Autodesk Fusion 360 part; units mm, degrees
note: some values were not read from the file. Set by a fixed rule: which sketch regions a step uses.
(part 2 of 3)
  measures "d194" angle of origin P53 P54
  measures "d195" angle of origin P53 P55
  measures "d196" distance of P52 P54
  measures "d198" distance of P52 L175
  measures "d200" distance of P53 L182
  measures "d202" distance of P54 L189
  measures "d204" distance of P55 L196
  measures "d205" diameter of A174
  measures "d206" diameter of A175
  measures "d207" distance of L158 A174.centre
  measures "d208" distance of L158 A175.centre
  measures "d211" diameter of A176
  measures "d212" diameter of A177
  measures "d213" distance of L154 A176.centre
  measures "d214" distance of L155 A177.centre
  measures "d215" vertical distance of A149.start A176.centre
  measures "d216" vertical distance of A142.end A177.centre
  measures "d217" diameter of A178
  measures "d218" diameter of A179
  measures "d219" diameter of A180
  measures "d220" diameter of A181
  measures "d221" diameter of A182
  measures "d222" diameter of A183
  measures "d223" distance of L108 A181.centre
  measures "d224" distance of L107 A180.centre
  measures "d225" distance of L114 A180.centre
  measures "d226" distance of L128 A181.centre
  measures "d229" diameter of A184
  measures "d230" diameter of A185
  measures "d231" radius of A187
  measures "d232" radius of A186
  measures "d233" radius of A188
  measures "d234" radius of A190
  measures "d235" radius of A193
  measures "d236" radius of A192
  measures "d237" radius of A196
  measures "d238" radius of A198
  measures "d240" distance of P56 L208
  measures "d242" distance of P57 L215
  measures "d246" distance of P58 L223
  measures "d247" distance of P59 L229
extrude "Extrude3" add sketch "Sketch1" along normal blind 4 contours A0 L17 L18 L19 L20 L21 L22 A11 A12 A13 | A0 L4 A3 L8 A4 L9 L16 L17 L18 L19 L20 L23 L24 L25 L26 L27 L28 A14 A15 A16 A17 A92 | A0 L4 A3 L9 L16 L19 | L27 L28 L33 L34 L59 L62 L82 L97 L99 L100 L101 L102 A82 A83 A84 A85 A86 A87 A88 A89 A90 A91 A92 A93 L103 L104 L105 L106 L107 L108 A114 A115 A116 A117 A118 A119 L140 A132 L143 A142 L145 A148 A149 L153 L154 L155 | L33 L34 L35 L36 A22 A23 L37 L38 A24 A25 L39 L40 A26 A27 L41 L42 A28 A93 | L55 L57 A46 A48 L65 L66 L74 A62 L82 A69 A72 L91 L93 A75 A81 L97 L98 A91 | A42 L59 L60 L61 L62 A49 L67 A51 L68 L75 L76 A60 L77 A61 L80 A64 A68 A90 | L158 A172 L192 L193 L194 L195 | L158 A172 L191 L192 L195 L196 | L170 L171 L172 L173 L174 L175 | L177 L178 L179 L180 L181 L182 | L184 L185 L186 L187 L188 L189 | A178 | A179 | A182 | A183 | A184 | A185 | L203 L204 L205 L206 L207 L208 | L210 L211 L212 L213 L214 L215 | L218 L219 L220 L221 L222 L223 | L224 L225 L226 L227 L228 L229 picked at (36.4142, -25.9017) picked at (-36.4142, 25.9017) picked at (-36.4142, -25.9017) makes body 1
extrude "Extrude4" cut sketch "Sketch1" along normal blind 2 contours L158 A172 L192 L193 L194 L195 | L158 A172 L191 L192 L195 L196 | A170 | L170 L171 L172 L173 L174 L175 | L177 L178 L179 L180 L181 L182 | L184 L185 L186 L187 L188 L189 | L203 L204 L205 L206 L207 L208 | L210 L211 L212 L213 L214 L215 | L218 L219 L220 L221 L222 L223 | L224 L225 L226 L227 L228 L229 bodies 1
extrude "Extrude5" cut sketch "Sketch1" against normal blind 1.425 draft 45 from surface at 1.425 contours A174 | A175 | A176 | A177 | A180 | A181 bodies 1
sketch "Sketch3" plane through (0, 0, 0) normal (0, 0, 1) x (1, 0, 0)
  circle A0 centre (-12.5, -19.2597) radius 3
  circle A1 centre (-12.5, -19.2597) radius 1.575
  circle A2 centre (12.5, -19.2597) radius 3
  circle A3 centre (12.5, -19.2597) radius 1.575
  circle A4 centre (-8.5, 32.168) radius 3
  circle A5 centre (-8.5, 32.168) radius 1.575
  circle A6 centre (8.5, 32.168) radius 3
  circle A7 centre (8.5, 32.168) radius 1.575
  line L0 (-11.5, -14.5484) -> (-15.5, -16.8578)
  line L1 (-11, -14.2597) -> (-5.2265, -14.2597) construction
  line L2 (-11.5, -23.971) -> (-15.5, -21.6616)
  line L3 (-11, -24.2597) -> (-5.2265, -24.2597) construction
  line L4 (11.5, -14.5484) -> (15.5, -16.8578)
  line L5 (11, -14.2597) -> (16.7735, -14.2597) construction
  line L6 (11.5, -23.971) -> (15.5, -21.6616)
  line L7 (-16, -17.7238) -> (-16, -20.7956)
  line L8 (16, -17.7238) -> (16, -20.7956)
  line L9 (-11, -24.837) -> (-11, -56.8259)
  line L10 (11, -56.8259) -> (11, -24.837)
  arc A8 (-11, -24.837) -> (-11.5, -23.971) centre (-12, -24.837) ccw
  arc A9 (11.5, -23.971) -> (11, -24.837) centre (12, -24.837) ccw
  arc A10 (15.5, -21.6616) -> (16, -20.7956) centre (15, -20.7956) ccw
  arc A11 (-16, -20.7956) -> (-15.5, -21.6616) centre (-15, -20.7956) ccw
  arc A12 (-15.5, -16.8578) -> (-16, -17.7238) centre (-15, -17.7238) ccw
  arc A13 (16, -17.7238) -> (15.5, -16.8578) centre (15, -17.7238) ccw
  arc A14 (11, -13.6823) -> (11.5, -14.5484) centre (12, -13.6823) ccw
  arc A15 (-11.5, -14.5484) -> (-11, -13.6823) centre (-12, -13.6823) ccw
  line L11 (-11, -56.8259) -> (-11, -57.116)
  line L12 (11, -56.8259) -> (11, -57.116)
  circle A16 centre (-6, -56) radius 3
  circle A17 centre (-6, -56) radius 1.575
  circle A18 centre (6, -56) radius 3
  circle A19 centre (6, -56) radius 1.575
  line L13 (-6, -56) -> (3.8151, -56) construction
  line L14 (6, -56) -> (15.3343, -56) construction
  line L15 (3.3188, -58.2498) -> (0.766, -55.2074)
  line L16 (-3.3188, -58.2498) -> (-0.766, -55.2074)
  arc A20 (-6.0502, -59.4996) -> (-3.3188, -58.2498) centre (-6, -56) ccw
  arc A21 (3.3188, -58.2498) -> (6.0502, -59.4996) centre (6, -56) ccw
  line L17 (6.7055, -59.3792) -> (10.342, -58.0557)
  line L18 (-10.342, -58.0557) -> (-6.7055, -59.3792)
  arc A22 (-11, -57.116) -> (-10.342, -58.0557) centre (-10, -57.116) ccw
  arc A23 (10.342, -58.0557) -> (11, -57.116) centre (10, -57.116) ccw
  arc A24 (0.766, -55.2074) -> (-0.766, -55.2074) centre (0, -55.8502) ccw
  arc A25 (-6.7055, -59.3792) -> (-6.0502, -59.4996) centre (-6.0215, -57.4998) ccw
  arc A26 (6.0502, -59.4996) -> (6.7055, -59.3792) centre (6.0215, -57.4998) ccw
  line L19 (-14.5, 29.0341) -> (-11.5, 27.302)
  line L20 (-11, 26.436) -> (-11, -13.6823)
  line L21 (-15, 36.168) -> (-15, 29.9001)
  arc A27 (-15, 29.9001) -> (-14.5, 29.0341) centre (-14, 29.9001) ccw
  arc A28 (-11, 26.436) -> (-11.5, 27.302) centre (-12, 26.436) ccw
  arc A29 (-14, 37.168) -> (-15, 36.168) centre (-14, 36.168) ccw
  line L22 (0, 2.5) -> (0, 20)
  line L23 (15, 36.168) -> (15, 29.9001)
  arc A30 (11.5, 27.302) -> (11, 26.436) centre (12, 26.436) ccw
  line L24 (14.5, 29.0341) -> (11.5, 27.302)
  arc A31 (14.5, 29.0341) -> (15, 29.9001) centre (14, 29.9001) ccw
  arc A32 (15, 36.168) -> (14, 37.168) centre (14, 36.168) ccw
  line L25 (11, 26.436) -> (11, -13.6823)
  line L26 (14, 37.168) -> (-14, 37.168)
  point P0 (-8.5, 32.168)
  point P1 (-8.5, 32.168)
  point P2 (-12.5, -19.2597)
  point P3 (12.5, -19.2597)
  dimension "d276" = 150
  dimension "d277" = 150
  dimension "d278" = 30
  dimension "d292" = 1
  dimension "d295" = 3.5
  dimension "d296" = 3.5
  dimension "d297" = 1
  dimension "d298" = 2
  dimension "d336" = 1
  constraint horizontal L1
  constraint horizontal L3
  constraint horizontal L5
  constraint vertical L7
  constraint coincident L3.start L2
  constraint coincident L3.start L9
  constraint tangent L2 A8
  constraint tangent L9 A8
  constraint tangent L6 A9
  constraint tangent L10 A9
  constraint equal A8 A9
  constraint tangent L8 A10
  constraint tangent L6 A10
  constraint equal A8 A10
  constraint tangent L2 A11
  constraint tangent L7 A11
  constraint equal A8 A11
  constraint tangent L0 A12
  constraint tangent L7 A12
  constraint equal A8 A12
  constraint tangent L4 A13
  constraint tangent L8 A13
  constraint equal A8 A13
  constraint coincident L5.start L4
  constraint tangent L4 A14
  constraint equal A8 A14
  constraint coincident L1.start L0
  constraint tangent L0 A15
  constraint equal A8 A15
  constraint parallel L9 L11
  constraint parallel L10 L12
  constraint horizontal L13
  constraint coincident A16.centre A17.centre
  constraint horizontal L14
  constraint coincident A18.centre A19.centre
  constraint tangent L11 A22
  constraint tangent L18 A22
  constraint tangent L12 A23
  constraint tangent L17 A23
  constraint equal A22 A23
  constraint tangent L15 A24
  constraint tangent L16 A24
  constraint equal A22 A24
  constraint tangent L18 A25
  constraint tangent A20 A25
  constraint tangent A21 A26
  constraint tangent L17 A26
  constraint equal A25 A26
  constraint tangent A15 L20
  constraint tangent L19 A27
  constraint tangent L21 A27
  constraint tangent L19 A28
  constraint tangent L20 A28
  constraint equal A27 A28
  constraint tangent L21 A29
  constraint equal A27 A29
  constraint symmetric L19.start L22 L24.start
  constraint symmetric L21.end L22 L23.end
  constraint symmetric A27 L22 A31
  constraint symmetric L19.end L22 A30.start
  constraint symmetric L20.start L22 A30.end
  constraint symmetric A28 L22 A30
  constraint symmetric A29.start L22 A32.end
  constraint symmetric L21.start L22 L23.start
  constraint symmetric A29 L22 A32
  constraint tangent A14 L25
  constraint tangent A29 L26
  measures "d276" angle of L0 L1
  measures "d277" angle of L2 L3
  measures "d278" angle of L4 L5
  measures "d292" radius of A8
  measures "d295" distance of A16.centre L16.start
  measures "d296" distance of A18.centre L15.start
  measures "d297" radius of A22
  measures "d298" radius of A25
  measures "d336" radius of A27
extrude "Extrude6" add sketch "Sketch3" along normal blind 4 from surface at 24 separate body contours A0 | A2 | A4 | A6 | L0 L2 L4 L6 L7 L8 L9 L10 A8 A9 A10 A11 A12 A13 A14 A15 L11 L12 L15 L16 A20 A21 L17 L18 A22 A23 A24 A25 A26 L19 L20 L21 A27 A28 A29 L23 A30 L24 A31 A32 L25 L26 | A16 | A18 makes body 2
extrude "Extrude7" cut 1 faces at (3.6667, -0.3096, 28) along direction (0, 0, -1) blind 2 on bodies 2 bodies 2
sketch "Sketch4" plane through (0, 0, 0) normal (1, 0, 0) x (0, 1, 0)
  line L0 (66.4049, 13.1472) -> (60.5972, 4.8528)
  line L1 (61.0301, 28.0017) -> (54.4692, 29.8895)
  line L2 (66.646, 14.9783) -> (62.3565, 26.7637)
  line L3 (53.2322, 29.8469) -> (37.168, 24)
  line L4 (58.9589, 4) -> (52, 4)
  line L5 (37.168, 24) -> (32.168, 24)
  line L6 (32.168, 24) -> (47.168, 24) construction
  arc A0 (62.3565, 26.7637) -> (61.0301, 28.0017) centre (60.4771, 26.0797) ccw
  arc A1 (66.4049, 13.1472) -> (66.646, 14.9783) centre (64.7666, 14.2943) ccw
  arc A2 (58.9589, 4) -> (60.5972, 4.8528) centre (58.9589, 6) ccw
  arc A3 (54.4692, 29.8895) -> (53.2322, 29.8469) centre (53.9162, 27.9675) ccw
  line L7 (32.168, 24) -> (35.9116, 10.0288)
  line L8 (36.0503, 9.5111) -> (48.3446, 9.5111) construction
  line L9 (52, 4) -> (42.3899, 4)
  line L10 (40.9757, 4.5858) -> (36.4293, 9.1322)
  arc A4 (40.9757, 4.5858) -> (42.3899, 4) centre (42.3899, 6) ccw
  arc A5 (35.9116, 10.0288) -> (36.4293, 9.1322) centre (37.8435, 10.5464) ccw
  line L11 (42.7183, 7.7929) -> (39.3778, 11.1334)
  line L12 (62.7914, 14.0886) -> (58.4766, 7.9264)
  line L13 (62.912, 15.0042) -> (59.5027, 24.371)
  line L14 (58.8395, 24.99) -> (55.247, 26.0237)
  line L15 (53.9705, 25.0627) -> (53.9705, 8.5)
  line L16 (50.4705, 8.5) -> (50.4705, 23.6889)
  line L17 (57.6574, 7.5) -> (54.9705, 7.5)
  line L18 (49.1285, 24.6286) -> (38.4432, 20.7395)
  line L19 (49.4705, 7.5) -> (43.4254, 7.5)
  arc A6 (55.247, 26.0237) -> (53.9705, 25.0627) centre (54.9705, 25.0627) ccw
  arc A7 (59.5027, 24.371) -> (58.8395, 24.99) centre (58.563, 24.029) ccw
  arc A8 (62.7914, 14.0886) -> (62.912, 15.0042) centre (61.9723, 14.6622) ccw
  arc A9 (57.6574, 7.5) -> (58.4766, 7.9264) centre (57.6574, 8.5) ccw
  arc A10 (53.9705, 8.5) -> (54.9705, 7.5) centre (54.9705, 8.5) ccw
  arc A11 (49.4705, 7.5) -> (50.4705, 8.5) centre (49.4705, 8.5) ccw
  arc A12 (42.7183, 7.7929) -> (43.4254, 7.5) centre (43.4254, 8.5) ccw
  arc A13 (39.119, 11.5817) -> (39.3778, 11.1334) centre (40.0849, 11.8405) ccw
  line L20 (37.7852, 19.7998) -> (37.7852, 16.6911)
  line L21 (37.8193, 16.4323) -> (39.119, 11.5817)
  arc A14 (50.4705, 23.6889) -> (49.1285, 24.6286) centre (49.4705, 23.6889) ccw
  arc A15 (38.4432, 20.7395) -> (37.7852, 19.7998) centre (38.7852, 19.7998) ccw
  arc A16 (37.7852, 16.6911) -> (37.8193, 16.4323) centre (38.7852, 16.6911) ccw
  point P0 (60, 4)
  point P1 (37.168, 24)
  point P2 (36.0503, 9.5111)
  dimension "d312" = 8
  dimension "d313" = 5
  dimension "d319" = 15
  dimension "d320" = 2
  dimension "d322" = 2
  dimension "d324" = 3.5
  dimension "d325" = 1
  dimension "d326" = 1
  dimension "d327" = 1
  constraint coincident P1 L3.end
  constraint horizontal L4
  constraint horizontal L5
  constraint horizontal L6
  constraint tangent L1 A0
  constraint tangent L2 A0
  constraint tangent L0 A1
  constraint tangent L2 A1
  constraint equal A0 A1
  constraint coincident P0 L0
  constraint coincident P0 L4
  constraint tangent L0 A2
  constraint tangent L4 A2
  constraint equal A0 A2
  constraint tangent L1 A3
  constraint tangent L3 A3
  constraint equal A0 A3
  constraint horizontal L8
  constraint coincident P2 L8.start
  constraint parallel L4 L9
  constraint tangent L9 A4
  constraint tangent L10 A4
  constraint tangent L10 A5
  constraint tangent L7 A5
  constraint equal A4 A5
  constraint perpendicular L15 L17
  constraint perpendicular L16 L19
  constraint tangent L14 A6
  constraint tangent L15 A6
  constraint tangent L13 A7
  constraint tangent L14 A7
  constraint equal A6 A7
  constraint tangent L12 A8
  constraint tangent L13 A8
  constraint equal A6 A8
  constraint tangent L12 A9
  constraint tangent L17 A9
  constraint equal A6 A9
  constraint tangent L15 A10
  constraint tangent L17 A10
  constraint equal A6 A10
  constraint tangent L16 A11
  constraint tangent L19 A11
  constraint tangent L11 A12
  constraint tangent L19 A12
  constraint equal A11 A12
  constraint tangent L11 A13
  constraint equal A11 A13
  constraint tangent A13 L21
  constraint tangent L16 A14
  constraint tangent L18 A14
  constraint tangent L18 A15
  constraint tangent L20 A15
  constraint equal A14 A15
  constraint tangent L20 A16
  constraint tangent L21 A16
  constraint equal A14 A16
  measures "d312" distance of P0 L4.end
  measures "d313" distance of P1 L5.end
  measures "d319" distance of L5.end P2
  measures "d320" radius of A0
  measures "d322" radius of A4
  measures "d324" distance of L15 L16
  measures "d325" radius of A6
  measures "d326" radius of A11
  measures "d327" radius of A14
extrude "Extrude8" add sketch "Sketch4" along normal blind 2.5 from surface at -13.75 separate body makes body 3
extrude "Extrude9" add sketch "Sketch4" against normal blind 2.5 from surface at 13.75 separate body makes body 4
sketch "Sketch5" plane through (0, 0, 24) normal (0, 0, 1) x (-1, 0, 0)
  line L0 (13.75, -37.168) -> (13.75, -32.168)
  line L1 (13.75, -32.168) -> (11.25, -32.168)
  line L2 (11.25, -32.168) -> (11.25, -37.168)
  line L3 (11.25, -37.168) -> (13.75, -37.168)
  line L4 (13.75, -32.168) -> (11.25, -32.168)
  line L5 (11.25, -32.168) -> (11.25, -36.168)
  line L6 (11.25, -36.168) -> (13.75, -36.168)
  line L7 (13.75, -36.168) -> (13.75, -32.168)
  line L8 (-13.75, -32.168) -> (-11.25, -32.168)
  line L9 (-11.25, -32.168) -> (-11.25, -36.168)
  line L10 (-11.25, -36.168) -> (-13.75, -36.168)
  line L11 (-13.75, -36.168) -> (-13.75, -32.168)
  line L12 (-11.1, -36.318) -> (-13.9, -36.318)
  line L13 (-13.9, -36.318) -> (-13.9, -32.018)
  line L14 (-13.9, -32.018) -> (-11.1, -32.018)
  line L15 (-11.1, -32.018) -> (-11.1, -36.318)
  line L16 (13.9, -32.018) -> (11.1, -32.018)
  line L17 (11.1, -32.018) -> (11.1, -36.318)
  line L18 (11.1, -36.318) -> (13.9, -36.318)
  line L19 (13.9, -36.318) -> (13.9, -32.018)
  dimension "d337" = 4
  dimension "d338" = 2.5
  dimension "d339" = 4
  dimension "d340" = -0.15
  dimension "d341" = 0.15
  constraint horizontal L4
  constraint vertical L5
  constraint horizontal L6
  constraint vertical L7
  constraint coincident L2 L5.end
  constraint coincident L0.end L1.start
  constraint horizontal L8
  constraint vertical L9
  constraint horizontal L10
  constraint vertical L11
  measures "d337" distance of L0.end L6.end
  measures "d338" distance of L8.start L8.end
  measures "d339" distance of L8.start L10.end
extrude "Extrude10" add sketch "Sketch5" along normal blind 2 contours L0 L1 L2 L4 L5 L6 L7 | L8 L9 L10 L11 bodies 3 4
extrude "Extrude11" cut sketch "Sketch5" along normal blind 2 contours L0 L1 L2 L4 L5 L6 L7 | L0 L1 L2 L4 L5 L7 L16 L17 L18 L19 | L0 L2 L6 L18 | L8 L9 L10 L11 | L12 L13 L14 L15 bodies 2
sketch "Sketch6" plane through (0, 0, 4) normal (0, 0, -1) x (1, 0, 0)
  line L0 (13.75, -58.9589) -> (13.75, -42.3899)
  line L1 (13.75, -42.3899) -> (11.25, -42.3899)
  line L2 (11.25, -42.3899) -> (11.25, -58.9589)
  line L3 (11.25, -58.9589) -> (13.75, -58.9589)
  line L4 (-13.75, -58.9589) -> (-11.25, -58.9589)
  line L5 (-11.25, -42.3899) -> (-13.75, -42.3899)
  line L6 (13.75, -54.9589) -> (11.25, -54.9589)
  line L7 (11.25, -54.9589) -> (11.25, -43.3899)
  line L8 (11.25, -43.3899) -> (13.75, -43.3899)
  line L9 (13.75, -43.3899) -> (13.75, -54.9589)
  line L10 (-11.25, -54.9589) -> (-13.75, -54.9589)
  line L11 (-11.25, -43.3899) -> (-13.75, -43.3899)
  line L12 (13.9, -43.2399) -> (13.9, -55.1089)
  line L13 (13.9, -55.1089) -> (11.1, -55.1089)
  line L14 (11.1, -55.1089) -> (11.1, -43.2399)
  line L15 (11.1, -43.2399) -> (13.9, -43.2399)
  line L16 (-11.25, -54.9589) -> (-11.25, -43.3899)
  line L17 (-13.75, -43.3899) -> (-13.75, -54.9589)
  line L18 (-13.9, -43.2399) -> (-13.9, -55.1089)
  line L19 (-11.1, -55.1089) -> (-13.9, -55.1089)
  line L20 (-11.1, -55.1089) -> (-11.1, -43.2399)
  line L21 (-11.1, -43.2399) -> (-13.9, -43.2399)
  dimension "d346" = 4
  dimension "d347" = 1
  dimension "d348" = 4
  dimension "d349" = 1
  dimension "d350" = -0.15
  dimension "d351" = -0.15
  constraint horizontal L6
  constraint vertical L7
  constraint horizontal L8
  constraint vertical L9
  constraint coincident L2 L7.end
  constraint coincident L0 L6.start
  constraint perpendicular L11 L16
  constraint perpendicular L10 L17
  measures "d346" distance of L3 L6
  measures "d347" distance of L1 L8
  measures "d348" distance of L4 L10
  measures "d349" distance of L5 L11
extrude "Extrude12" add sketch "Sketch6" along normal blind 4 contours L0 L2 L6 L7 L8 L9 | L10 L11 L16 L17 bodies 3 4
extrude "Extrude13" cut sketch "Sketch6" along normal blind 4 contours L0 L2 L6 L7 L8 L9 | L0 L9 L12 L13 L15 | L0 L2 L6 L13 | L0 L2 L8 L15 | L2 L7 L13 L14 L15 | L10 L11 L16 L17 | L18 L19 L20 L21 bodies 1
extrude "Extrude14" cut sketch "Sketch3" along normal blind 1.425 draft 45 from surface at 24.575 contours A1 | A3 | A5 | A7 | A17 | A19 bodies 2 3 4
sketch "Sketch7" plane through (0, 0, 4) normal (0, 0, 1) x (-1, 0, 0)
  line L0 (-13.9, -43.2399) -> (-11.1, -43.2399)
  line L1 (-11.1, -43.2399) -> (-11.1, -55.1089)
  line L2 (-11.1, -55.1089) -> (-13.9, -55.1089)
  line L3 (-13.9, -55.1089) -> (-13.9, -43.2399)
  line L4 (13.9, -55.1089) -> (11.1, -55.1089)
  line L5 (11.1, -55.1089) -> (11.1, -43.2399)
  line L6 (11.1, -43.2399) -> (13.9, -43.2399)
  line L7 (13.9, -43.2399) -> (13.9, -55.1089)
  arc A0 (60.7453, -47.0282) -> (58.5719, -47.3691) centre (59.6586, -47.1987) ccw
  line L8 (60.7453, -47.0282) -> (61.032, -48.8558)
  arc A1 (58.8586, -49.1968) -> (61.032, -48.8558) centre (59.9453, -49.0263) ccw
  line L9 (58.8586, -49.1968) -> (58.5719, -47.3691)
  line L10 (-61.032, -48.8558) -> (-60.7453, -47.0282)
  arc A2 (-58.5719, -47.3691) -> (-60.7453, -47.0282) centre (-59.6586, -47.1987) ccw
  line L11 (-58.5719, -47.3691) -> (-58.8586, -49.1968)
  arc A3 (-61.032, -48.8558) -> (-58.8586, -49.1968) centre (-59.9453, -49.0263) ccw
  circle A4 centre (-10, 29.345) radius 1
  arc A5 (68.1327, -45.1089) -> (66.7394, -44.3498) centre (67.1447, -45.2639) ccw
  line L12 (68.1327, -45.1089) -> (68.783, -49.255)
  arc A6 (67.9501, -50.3979) -> (68.783, -49.255) centre (67.7951, -49.41) ccw
  line L13 (67.9501, -50.3979) -> (63.804, -51.0483)
  arc A7 (62.6547, -49.9543) -> (63.804, -51.0483) centre (63.649, -50.0604) ccw
  line L14 (62.6547, -49.9543) -> (63.0179, -46.547)
  arc A8 (63.6069, -45.7389) -> (63.0179, -46.547) centre (64.0123, -46.653) ccw
  line L15 (63.6069, -45.7389) -> (66.7394, -44.3498)
  arc A9 (8.2929, -47.4122) -> (10, -46.7051) centre (9, -46.7051) ccw
  line L16 (8.2929, -47.4122) -> (1.2929, -40.4122)
  arc A10 (1, -39.7051) -> (1.2929, -40.4122) centre (2, -39.7051) ccw
  line L17 (1, -39.7051) -> (1, -33.918)
  arc A11 (2, -32.918) -> (1, -33.918) centre (2, -33.918) ccw
  line L18 (2, -32.918) -> (3.6847, -32.918)
  arc A12 (4.2583, -33.0989) -> (3.6847, -32.918) centre (3.6847, -33.918) ccw
  line L19 (4.2583, -33.0989) -> (9.5736, -36.8207)
  arc A13 (10, -37.6399) -> (9.5736, -36.8207) centre (9, -37.6399) ccw
  line L20 (10, -37.6399) -> (10, -46.7051)
  circle A14 centre (18.0312, 0) radius 1.075
  arc A15 (65.1968, -43.1414) -> (64.8558, -40.968) centre (65.0263, -42.0547) ccw
  line L21 (65.1968, -43.1414) -> (63.3691, -43.4281)
  arc A16 (63.0282, -41.2547) -> (63.3691, -43.4281) centre (63.1987, -42.3414) ccw
  line L22 (63.0282, -41.2547) -> (64.8558, -40.968)
  circle A17 centre (-8.5, -32.168) radius 1.575
  circle A18 centre (-59, 43) radius 2.25
  arc A19 (-68.1327, 45.1089) -> (-66.7394, 44.3498) centre (-67.1447, 45.2639) ccw
  line L23 (-68.1327, 45.1089) -> (-68.783, 49.255)
  arc A20 (-67.9501, 50.3979) -> (-68.783, 49.255) centre (-67.7951, 49.41) ccw
  line L24 (-67.9501, 50.3979) -> (-63.804, 51.0483)
  arc A21 (-62.6547, 49.9543) -> (-63.804, 51.0483) centre (-63.649, 50.0604) ccw
  line L25 (-62.6547, 49.9543) -> (-63.0179, 46.547)
  arc A22 (-63.6069, 45.7389) -> (-63.0179, 46.547) centre (-64.0123, 46.653) ccw
  line L26 (-63.6069, 45.7389) -> (-66.7394, 44.3498)
  circle A23 centre (59, -43) radius 2.25
  line L27 (59.4281, 38.6309) -> (59.1414, 36.8032)
  arc A24 (56.968, 37.1442) -> (59.1414, 36.8032) centre (58.0547, 36.9737) ccw
  line L28 (56.968, 37.1442) -> (57.2547, 38.9718)
  arc A25 (59.4281, 38.6309) -> (57.2547, 38.9718) centre (58.3414, 38.8013) ccw
  line L29 (64.8558, 40.968) -> (63.0282, 41.2547)
  arc A26 (63.3691, 43.4281) -> (63.0282, 41.2547) centre (63.1987, 42.3414) ccw
  line L30 (63.3691, 43.4281) -> (65.1968, 43.1414)
  arc A27 (64.8558, 40.968) -> (65.1968, 43.1414) centre (65.0263, 42.0547) ccw
  arc A28 (-8.2929, -16.9667) -> (-10, -17.6738) centre (-9, -17.6738) ccw
  line L31 (-8.2929, -16.9667) -> (-1.2929, -23.9667)
  arc A29 (-1, -24.6738) -> (-1.2929, -23.9667) centre (-2, -24.6738) ccw
  line L32 (-1, -24.6738) -> (-1, -30.4608)
  arc A30 (-2, -31.4608) -> (-1, -30.4608) centre (-2, -30.4608) ccw
  line L33 (-2, -31.4608) -> (-3.6847, -31.4608)
  arc A31 (-4.2583, -31.2799) -> (-3.6847, -31.4608) centre (-3.6847, -30.4608) ccw
  line L34 (-4.2583, -31.2799) -> (-9.5736, -27.5581)
  arc A32 (-10, -26.739) -> (-9.5736, -27.5581) centre (-9, -26.739) ccw
  line L35 (-10, -26.739) -> (-10, -17.6738)
  line L36 (68.783, 49.255) -> (68.1327, 45.1089)
  arc A33 (66.7394, 44.3498) -> (68.1327, 45.1089) centre (67.1447, 45.2639) ccw
  line L37 (66.7394, 44.3498) -> (63.6069, 45.7389)
  arc A34 (63.0179, 46.547) -> (63.6069, 45.7389) centre (64.0123, 46.653) ccw
  line L38 (63.0179, 46.547) -> (62.6547, 49.9543)
  arc A35 (63.804, 51.0483) -> (62.6547, 49.9543) centre (63.649, 50.0604) ccw
  line L39 (63.804, 51.0483) -> (67.9501, 50.3979)
  arc A36 (68.783, 49.255) -> (67.9501, 50.3979) centre (67.7951, 49.41) ccw
  circle A37 centre (10, 49.345) radius 1
  arc A38 (-9.2448, 26.3539) -> (-10, 25.3844) centre (-9, 25.3844) ccw
  arc A39 (-9.2448, 26.3539) -> (-6.935, 28.9943) centre (-10, 29.345) ccw
  arc A40 (-6.5151, 29.6997) -> (-6.935, 28.9943) centre (-5.9415, 28.8805) ccw
  line L40 (-6.5151, 29.6997) -> (-4.2583, 31.2799)
  arc A41 (-3.6847, 31.4608) -> (-4.2583, 31.2799) centre (-3.6847, 30.4608) ccw
  line L41 (-3.6847, 31.4608) -> (-2, 31.4608)
  arc A42 (-1, 30.4608) -> (-2, 31.4608) centre (-2, 30.4608) ccw
  line L42 (-1, 30.4608) -> (-1, 24.6738)
  arc A43 (-1.2929, 23.9667) -> (-1, 24.6738) centre (-2, 24.6738) ccw
  line L43 (-1.2929, 23.9667) -> (-8.2929, 16.9667)
  arc A44 (-9.1655, 16.6876) -> (-8.2929, 16.9667) centre (-9, 17.6738) ccw
  arc A45 (-9.5099, 17.4405) -> (-9.1655, 16.6876) centre (-9.0827, 17.1807) ccw
  arc A46 (-9.5099, 17.4405) -> (-9.7778, 21.4596) centre (-12.5, 19.2597) ccw
  arc A47 (-10, 22.0881) -> (-9.7778, 21.4596) centre (-9, 22.0881) ccw
  line L44 (-10, 22.0881) -> (-10, 25.3844)
  circle A48 centre (6, 56) radius 1.575
  arc A49 (-59.1414, 36.8032) -> (-56.968, 37.1442) centre (-58.0547, 36.9737) ccw
  line L45 (-59.1414, 36.8032) -> (-59.4281, 38.6309)
  arc A50 (-57.2547, 38.9718) -> (-59.4281, 38.6309) centre (-58.3414, 38.8013) ccw
  line L46 (-57.2547, 38.9718) -> (-56.968, 37.1442)
  arc A51 (9.5736, 36.8207) -> (10, 37.6399) centre (9, 37.6399) ccw
  line L47 (9.5736, 36.8207) -> (4.2583, 33.0989)
  arc A52 (3.6847, 32.918) -> (4.2583, 33.0989) centre (3.6847, 33.918) ccw
  line L48 (3.6847, 32.918) -> (2, 32.918)
  arc A53 (1, 33.918) -> (2, 32.918) centre (2, 33.918) ccw
  line L49 (1, 33.918) -> (1, 39.7051)
  arc A54 (1.2929, 40.4122) -> (1, 39.7051) centre (2, 39.7051) ccw
  line L50 (1.2929, 40.4122) -> (7.4059, 46.5252)
  arc A55 (8.5848, 46.6998) -> (7.4059, 46.5252) centre (8.113, 45.8181) ccw
  arc A56 (8.5848, 46.6998) -> (9.25, 46.4403) centre (10, 49.345) ccw
  arc A57 (10, 45.472) -> (9.25, 46.4403) centre (9, 45.472) ccw
  line L51 (10, 45.472) -> (10, 37.6399)
  circle A58 centre (59, 43) radius 2.25
  circle A59 centre (-6, 56) radius 1.575
  arc A60 (-63.0179, -46.547) -> (-63.6069, -45.7389) centre (-64.0123, -46.653) ccw
  line L52 (-63.0179, -46.547) -> (-62.6547, -49.9543)
  arc A61 (-63.804, -51.0483) -> (-62.6547, -49.9543) centre (-63.649, -50.0604) ccw
  line L53 (-63.804, -51.0483) -> (-67.9501, -50.3979)
  arc A62 (-68.783, -49.255) -> (-67.9501, -50.3979) centre (-67.7951, -49.41) ccw
  line L54 (-68.783, -49.255) -> (-68.1327, -45.1089)
  arc A63 (-66.7394, -44.3498) -> (-68.1327, -45.1089) centre (-67.1447, -45.2639) ccw
  line L55 (-66.7394, -44.3498) -> (-63.6069, -45.7389)
  circle A64 centre (12.5, 19.2597) radius 1.575
  line L56 (-53.1442, -45.032) -> (-54.9718, -44.7453)
  arc A65 (-54.6309, -42.5719) -> (-54.9718, -44.7453) centre (-54.8013, -43.6586) ccw
  line L57 (-54.6309, -42.5719) -> (-52.8032, -42.8586)
  arc A66 (-53.1442, -45.032) -> (-52.8032, -42.8586) centre (-52.9737, -43.9453) ccw
  line L58 (-59.4281, -38.6309) -> (-59.1414, -36.8032)
  arc A67 (-56.968, -37.1442) -> (-59.1414, -36.8032) centre (-58.0547, -36.9737) ccw
  line L59 (-56.968, -37.1442) -> (-57.2547, -38.9718)
  arc A68 (-59.4281, -38.6309) -> (-57.2547, -38.9718) centre (-58.3414, -38.8013) ccw
  circle A69 centre (-12.5, 19.2597) radius 1.575
  arc A70 (8.2929, 16.9667) -> (9.1655, 16.6876) centre (9, 17.6738) ccw
  line L60 (8.2929, 16.9667) -> (1.2929, 23.9667)
  arc A71 (1, 24.6738) -> (1.2929, 23.9667) centre (2, 24.6738) ccw
  line L61 (1, 24.6738) -> (1, 30.4608)
  arc A72 (2, 31.4608) -> (1, 30.4608) centre (2, 30.4608) ccw
  line L62 (2, 31.4608) -> (3.6847, 31.4608)
  arc A73 (4.2583, 31.2799) -> (3.6847, 31.4608) centre (3.6847, 30.4608) ccw
  line L63 (4.2583, 31.2799) -> (6.5151, 29.6997)
  arc A74 (6.935, 28.9943) -> (6.5151, 29.6997) centre (5.9415, 28.8805) ccw
  arc A75 (6.935, 28.9943) -> (9.2448, 26.3539) centre (10, 29.345) ccw
  arc A76 (10, 25.3844) -> (9.2448, 26.3539) centre (9, 25.3844) ccw
  line L64 (10, 25.3844) -> (10, 22.0881)
  arc A77 (9.7778, 21.4596) -> (10, 22.0881) centre (9, 22.0881) ccw
  arc A78 (9.7778, 21.4596) -> (9.5099, 17.4405) centre (12.5, 19.2597) ccw
  arc A79 (9.1655, 16.6876) -> (9.5099, 17.4405) centre (9.0827, 17.1807) ccw
  line L65 (53.1442, 45.032) -> (54.9718, 44.7453)
  arc A80 (54.6309, 42.5719) -> (54.9718, 44.7453) centre (54.8013, 43.6586) ccw
  line L66 (54.6309, 42.5719) -> (52.8032, 42.8586)
  arc A81 (53.1442, 45.032) -> (52.8032, 42.8586) centre (52.9737, 43.9453) ccw
  arc A82 (-9.5736, -36.8207) -> (-10, -37.6399) centre (-9, -37.6399) ccw
  line L67 (-9.5736, -36.8207) -> (-4.2583, -33.0989)
  arc A83 (-3.6847, -32.918) -> (-4.2583, -33.0989) centre (-3.6847, -33.918) ccw
  line L68 (-3.6847, -32.918) -> (-2, -32.918)
  arc A84 (-1, -33.918) -> (-2, -32.918) centre (-2, -33.918) ccw
  line L69 (-1, -33.918) -> (-1, -39.7051)
  arc A85 (-1.2929, -40.4122) -> (-1, -39.7051) centre (-2, -39.7051) ccw
  line L70 (-1.2929, -40.4122) -> (-8.2929, -47.4122)
  arc A86 (-10, -46.7051) -> (-8.2929, -47.4122) centre (-9, -46.7051) ccw
  line L71 (-10, -46.7051) -> (-10, -37.6399)
  circle A87 centre (-10, 49.345) radius 1
  circle A88 centre (10, 29.345) radius 1
  arc A89 (10, -17.6738) -> (8.2929, -16.9667) centre (9, -17.6738) ccw
  line L72 (10, -17.6738) -> (10, -26.739)
  arc A90 (9.5736, -27.5581) -> (10, -26.739) centre (9, -26.739) ccw
  line L73 (9.5736, -27.5581) -> (4.2583, -31.2799)
  arc A91 (3.6847, -31.4608) -> (4.2583, -31.2799) centre (3.6847, -30.4608) ccw
  line L74 (3.6847, -31.4608) -> (2, -31.4608)
  arc A92 (1, -30.4608) -> (2, -31.4608) centre (2, -30.4608) ccw
  line L75 (1, -30.4608) -> (1, -24.6738)
  arc A93 (1.2929, -23.9667) -> (1, -24.6738) centre (2, -24.6738) ccw
  line L76 (1.2929, -23.9667) -> (8.2929, -16.9667)
  circle A94 centre (8.5, -32.168) radius 1.575
  arc A95 (52.8032, -42.8586) -> (53.1442, -45.032) centre (52.9737, -43.9453) ccw
  line L77 (52.8032, -42.8586) -> (54.6309, -42.5719)
  arc A96 (54.9718, -44.7453) -> (54.6309, -42.5719) centre (54.8013, -43.6586) ccw
  line L78 (54.9718, -44.7453) -> (53.1442, -45.032)
  circle A97 centre (-59, -43) radius 2.25
  circle A98 centre (-18.0312, 0) radius 1.075
  line L79 (4.1184, -55.5) -> (-4.1184, -55.5)
  arc A99 (-5.8285, -55.1985) -> (-4.1184, -55.5) centre (-4.1184, -50.5) ccw
  line L80 (-5.8285, -55.1985) -> (-9.342, -53.9196)
  arc A100 (-10, -52.9799) -> (-9.342, -53.9196) centre (-9, -52.9799) ccw
  line L81 (-10, -52.9799) -> (-10, -51.5944)
  arc A101 (-9.7071, -50.8873) -> (-10, -51.5944) centre (-9, -51.5944) ccw
  line L82 (-9.7071, -50.8873) -> (-0.7071, -41.8873)
  arc A102 (0.7071, -41.8873) -> (-0.7071, -41.8873) centre (0, -42.5944) ccw
  line L83 (0.7071, -41.8873) -> (9.7071, -50.8873)
  arc A103 (10, -51.5944) -> (9.7071, -50.8873) centre (9, -51.5944) ccw
  line L84 (10, -51.5944) -> (10, -52.9799)
  arc A104 (9.342, -53.9196) -> (10, -52.9799) centre (9, -52.9799) ccw
  line L85 (9.342, -53.9196) -> (5.8285, -55.1985)
  arc A105 (4.1184, -55.5) -> (5.8285, -55.1985) centre (4.1184, -50.5) ccw
  arc A106 (-63.0282, 41.2547) -> (-63.3691, 43.4281) centre (-63.1987, 42.3414) ccw
  line L86 (-63.0282, 41.2547) -> (-64.8558, 40.968)
  arc A107 (-65.1968, 43.1414) -> (-64.8558, 40.968) centre (-65.0263, 42.0547) ccw
  line L87 (-65.1968, 43.1414) -> (-63.3691, 43.4281)
  arc A108 (-9.25, 46.4403) -> (-10, 45.472) centre (-9, 45.472) ccw
  arc A109 (-9.25, 46.4403) -> (-8.5848, 46.6998) centre (-10, 49.345) ccw
  arc A110 (-7.4059, 46.5252) -> (-8.5848, 46.6998) centre (-8.113, 45.8181) ccw
  line L88 (-7.4059, 46.5252) -> (-1.2929, 40.4122)
  arc A111 (-1, 39.7051) -> (-1.2929, 40.4122) centre (-2, 39.7051) ccw
  line L89 (-1, 39.7051) -> (-1, 33.918)
  arc A112 (-2, 32.918) -> (-1, 33.918) centre (-2, 33.918) ccw
  line L90 (-2, 32.918) -> (-3.6847, 32.918)
  arc A113 (-4.2583, 33.0989) -> (-3.6847, 32.918) centre (-3.6847, 33.918) ccw
  line L91 (-4.2583, 33.0989) -> (-9.5736, 36.8207)
  arc A114 (-10, 37.6399) -> (-9.5736, 36.8207) centre (-9, 37.6399) ccw
  line L92 (-10, 37.6399) -> (-10, 45.472)
  arc A115 (61.032, 48.8558) -> (58.8586, 49.1968) centre (59.9453, 49.0263) ccw
  line L93 (61.032, 48.8558) -> (60.7453, 47.0282)
  arc A116 (58.5719, 47.3691) -> (60.7453, 47.0282) centre (59.6586, 47.1987) ccw
  line L94 (58.5719, 47.3691) -> (58.8586, 49.1968)
  circle A117 centre (0, 18.0312) radius 1.075
  circle A118 centre (0, -18.0312) radius 1.075
  arc A119 (-60.7453, 47.0282) -> (-58.5719, 47.3691) centre (-59.6586, 47.1987) ccw
  line L95 (-60.7453, 47.0282) -> (-61.032, 48.8558)
  arc A120 (-58.8586, 49.1968) -> (-61.032, 48.8558) centre (-59.9453, 49.0263) ccw
  line L96 (-58.8586, 49.1968) -> (-58.5719, 47.3691)
  line L97 (-64.8558, -40.968) -> (-63.0282, -41.2547)
  arc A121 (-63.3691, -43.4281) -> (-63.0282, -41.2547) centre (-63.1987, -42.3414) ccw
  line L98 (-63.3691, -43.4281) -> (-65.1968, -43.1414)
  arc A122 (-64.8558, -40.968) -> (-65.1968, -43.1414) centre (-65.0263, -42.0547) ccw
  arc A123 (9.2732, 53.9447) -> (8.7144, 53.7905) centre (9.1022, 53.4748) ccw
  line L99 (9.2732, 53.9447) -> (9.342, 53.9196)
  arc A124 (10, 52.9799) -> (9.342, 53.9196) centre (9, 52.9799) ccw
  line L100 (10, 52.9799) -> (10, 52.8091)
  arc A125 (9.5714, 52.3143) -> (10, 52.8091) centre (9.5, 52.8091) ccw
  arc A126 (9.5714, 52.3143) -> (7.045, 48.8271) centre (10, 49.345) ccw
  arc A127 (6.7672, 47.9473) -> (7.045, 48.8271) centre (6.0601, 48.6544) ccw
  line L101 (6.7672, 47.9473) -> (0.7071, 41.8873)
  arc A128 (-0.7071, 41.8873) -> (0.7071, 41.8873) centre (0, 42.5944) ccw
  line L102 (-0.7071, 41.8873) -> (-6.7672, 47.9473)
  arc A129 (-7.045, 48.8271) -> (-6.7672, 47.9473) centre (-6.0601, 48.6544) ccw
  arc A130 (-7.045, 48.8271) -> (-9.5714, 52.3143) centre (-10, 49.345) ccw
  arc A131 (-10, 52.8091) -> (-9.5714, 52.3143) centre (-9.5, 52.8091) ccw
  line L103 (-10, 52.8091) -> (-10, 52.9799)
  arc A132 (-9.342, 53.9196) -> (-10, 52.9799) centre (-9, 52.9799) ccw
  line L104 (-9.342, 53.9196) -> (-9.2732, 53.9447)
  arc A133 (-8.7144, 53.7905) -> (-9.2732, 53.9447) centre (-9.1022, 53.4748) ccw
  arc A134 (-8.7144, 53.7905) -> (-2.7002, 54.8333) centre (-6, 56) ccw
  arc A135 (-1.7574, 55.5) -> (-2.7002, 54.8333) centre (-1.7574, 54.5) ccw
  line L105 (-1.7574, 55.5) -> (1.7574, 55.5)
  arc A136 (2.7002, 54.8333) -> (1.7574, 55.5) centre (1.7574, 54.5) ccw
  arc A137 (2.7002, 54.8333) -> (8.7144, 53.7905) centre (6, 56) ccw
  arc A138 (59.1414, -36.8032) -> (56.968, -37.1442) centre (58.0547, -36.9737) ccw
  line L106 (59.1414, -36.8032) -> (59.4281, -38.6309)
  arc A139 (57.2547, -38.9718) -> (59.4281, -38.6309) centre (58.3414, -38.8013) ccw
  line L107 (57.2547, -38.9718) -> (56.968, -37.1442)
  arc A140 (-54.9718, 44.7453) -> (-54.6309, 42.5719) centre (-54.8013, 43.6586) ccw
  line L108 (-54.9718, 44.7453) -> (-53.1442, 45.032)
  arc A141 (-52.8032, 42.8586) -> (-53.1442, 45.032) centre (-52.9737, 43.9453) ccw
  line L109 (-52.8032, 42.8586) -> (-54.6309, 42.5719)
  line L110 (4.1184, 60) -> (-4.1184, 60)
  arc A142 (-4.1184, 60) -> (-5.8285, 59.6985) centre (-4.1184, 55) ccw
  line L111 (-5.8285, 59.6985) -> (-13.0261, 57.0788)
  arc A143 (-13.0261, 57.0788) -> (-15, 54.2597) centre (-12, 54.2597) ccw
  line L112 (-15, 54.2597) -> (-15, 22.432)
  arc A144 (-18.7908, 20.291) -> (-15, 22.432) centre (-17.5, 22.432) ccw
  line L113 (-18.7908, 20.291) -> (-38.0643, 31.9107)
  line L114 (-38.0643, 31.9107) -> (-43.3688, 35.7766)
  arc A145 (-47.8072, 40.8084) -> (-43.3688, 35.7766) centre (-34.2395, 48.3029) ccw
  line L115 (-47.8072, 40.8084) -> (-49.7459, 44.3181)
  arc A146 (-49.7459, 44.3181) -> (-50.4618, 45.1297) centre (-51.9342, 43.1093) ccw
  line L116 (-50.4618, 45.1297) -> (-60.6297, 52.5402)
  arc A147 (-60.6297, 52.5402) -> (-63.9775, 53.3492) centre (-63.2801, 48.9036) ccw
  line L117 (-63.9775, 53.3492) -> (-70.0847, 52.3912)
  arc A148 (-70.0847, 52.3912) -> (-71.3342, 50.6769) centre (-69.8523, 50.9093) ccw
  line L118 (-71.3342, 50.6769) -> (-70.3762, 44.5696)
  arc A149 (-70.3762, 44.5696) -> (-68.581, 41.6303) centre (-65.9305, 45.2669) ccw
  line L119 (-68.581, 41.6303) -> (-58.4131, 34.2198)
  arc A150 (-58.4131, 34.2198) -> (-57.4213, 33.7868) centre (-56.9406, 36.2401) ccw
  line L120 (-57.4213, 33.7868) -> (-53.4866, 33.0159)
  arc A151 (-47.3374, 30.3313) -> (-53.4866, 33.0159) centre (-56.4667, 17.8051) ccw
  line L121 (-47.3374, 30.3313) -> (-42.033, 26.4653)
  line L122 (-42.033, 26.4653) -> (-18.153, 5.6444)
  arc A152 (-18.0781, 3.4531) -> (-18.153, 5.6444) centre (-19.1387, 4.5138) ccw
  line L123 (-18.0781, 3.4531) -> (-19.7635, 1.7678)
  arc A153 (-19.7635, 1.7678) -> (-19.7635, -1.7678) centre (-17.9957, 0) ccw
  line L124 (-19.7635, -1.7678) -> (-18.0781, -3.4531)
  arc A154 (-18.153, -5.6444) -> (-18.0781, -3.4531) centre (-19.1387, -4.5138) ccw
  line L125 (-18.153, -5.6444) -> (-42.033, -26.4653)
  line L126 (-42.033, -26.4653) -> (-47.3374, -30.3313)
  arc A155 (-53.4866, -33.0159) -> (-47.3374, -30.3313) centre (-56.4667, -17.8051) ccw
  line L127 (-53.4866, -33.0159) -> (-57.4213, -33.7868)
  arc A156 (-57.4213, -33.7868) -> (-58.4131, -34.2198) centre (-56.9406, -36.2401) ccw
  line L128 (-58.4131, -34.2198) -> (-68.581, -41.6303)
  arc A157 (-68.581, -41.6303) -> (-70.3762, -44.5696) centre (-65.9305, -45.2669) ccw
  line L129 (-70.3762, -44.5696) -> (-71.3342, -50.6769)
  arc A158 (-71.3342, -50.6769) -> (-70.0847, -52.3912) centre (-69.8523, -50.9093) ccw
  line L130 (-70.0847, -52.3912) -> (-63.9775, -53.3492)
  arc A159 (-63.9775, -53.3492) -> (-60.6297, -52.5402) centre (-63.2801, -48.9036) ccw
  line L131 (-60.6297, -52.5402) -> (-50.4618, -45.1297)
  arc A160 (-50.4618, -45.1297) -> (-49.7459, -44.3181) centre (-51.9342, -43.1093) ccw
  line L132 (-49.7459, -44.3181) -> (-47.8072, -40.8084)
  arc A161 (-43.3688, -35.7766) -> (-47.8072, -40.8084) centre (-34.2395, -48.3029) ccw
  line L133 (-43.3688, -35.7766) -> (-38.0643, -31.9107)
  line L134 (-38.0643, -31.9107) -> (-18.7908, -20.291)
  arc A162 (-15, -22.432) -> (-18.7908, -20.291) centre (-17.5, -22.432) ccw
  line L135 (-15, -22.432) -> (-15, -54.2597)
  arc A163 (-15, -54.2597) -> (-13.0261, -57.0788) centre (-12, -54.2597) ccw
  line L136 (-13.0261, -57.0788) -> (-5.8285, -59.6985)
  arc A164 (-5.8285, -59.6985) -> (-4.1184, -60) centre (-4.1184, -55) ccw
  line L137 (-4.1184, -60) -> (4.1184, -60)
  arc A165 (4.1184, -60) -> (5.8285, -59.6985) centre (4.1184, -55) ccw
  line L138 (5.8285, -59.6985) -> (13.0261, -57.0788)
  arc A166 (13.0261, -57.0788) -> (15, -54.2597) centre (12, -54.2597) ccw
  line L139 (15, -54.2597) -> (15, -22.432)
  arc A167 (18.7908, -20.291) -> (15, -22.432) centre (17.5, -22.432) ccw
  line L140 (18.7908, -20.291) -> (38.0643, -31.9107)
  line L141 (38.0643, -31.9107) -> (43.3688, -35.7766)
  arc A168 (47.8072, -40.8084) -> (43.3688, -35.7766) centre (34.2395, -48.3029) ccw
  line L142 (47.8072, -40.8084) -> (49.7459, -44.3181)
  arc A169 (49.7459, -44.3181) -> (50.4618, -45.1297) centre (51.9342, -43.1093) ccw
  line L143 (50.4618, -45.1297) -> (60.6297, -52.5402)
  arc A170 (60.6297, -52.5402) -> (63.9775, -53.3492) centre (63.2801, -48.9036) ccw
  line L144 (63.9775, -53.3492) -> (70.0847, -52.3912)
  arc A171 (70.0847, -52.3912) -> (71.3342, -50.6769) centre (69.8523, -50.9093) ccw
  line L145 (71.3342, -50.6769) -> (70.3762, -44.5696)
  arc A172 (70.3762, -44.5696) -> (68.581, -41.6303) centre (65.9305, -45.2669) ccw
  line L146 (68.581, -41.6303) -> (58.4131, -34.2198)
  arc A173 (58.4131, -34.2198) -> (57.4213, -33.7868) centre (56.9406, -36.2401) ccw
  line L147 (57.4213, -33.7868) -> (53.4866, -33.0159)
  arc A174 (47.3374, -30.3313) -> (53.4866, -33.0159) centre (56.4667, -17.8051) ccw
  line L148 (47.3374, -30.3313) -> (42.033, -26.4653)
  line L149 (42.033, -26.4653) -> (18.153, -5.6444)
  arc A175 (18.0781, -3.4531) -> (18.153, -5.6444) centre (19.1387, -4.5138) ccw
  line L150 (18.0781, -3.4531) -> (19.7635, -1.7678)
  arc A176 (19.7635, -1.7678) -> (19.7635, 1.7678) centre (17.9957, 0) ccw
  line L151 (19.7635, 1.7678) -> (18.0781, 3.4531)
  arc A177 (18.153, 5.6444) -> (18.0781, 3.4531) centre (19.1387, 4.5138) ccw
  line L152 (18.153, 5.6444) -> (42.033, 26.4653)
  line L153 (42.033, 26.4653) -> (47.3374, 30.3313)
  arc A178 (53.4866, 33.0159) -> (47.3374, 30.3313) centre (56.4667, 17.8051) ccw
  line L154 (53.4866, 33.0159) -> (57.4213, 33.7868)
  arc A179 (57.4213, 33.7868) -> (58.4131, 34.2198) centre (56.9406, 36.2401) ccw
  line L155 (58.4131, 34.2198) -> (68.581, 41.6303)
  arc A180 (68.581, 41.6303) -> (70.3762, 44.5696) centre (65.9305, 45.2669) ccw
  line L156 (70.3762, 44.5696) -> (71.3342, 50.6769)
  arc A181 (71.3342, 50.6769) -> (70.0847, 52.3912) centre (69.8523, 50.9093) ccw
  line L157 (70.0847, 52.3912) -> (63.9775, 53.3492)
  arc A182 (63.9775, 53.3492) -> (60.6297, 52.5402) centre (63.2801, 48.9036) ccw
  line L158 (60.6297, 52.5402) -> (50.4618, 45.1297)
  arc A183 (50.4618, 45.1297) -> (49.7459, 44.3181) centre (51.9342, 43.1093) ccw
  line L159 (49.7459, 44.3181) -> (47.8072, 40.8084)
  arc A184 (43.3688, 35.7766) -> (47.8072, 40.8084) centre (34.2395, 48.3029) ccw
  line L160 (43.3688, 35.7766) -> (38.0643, 31.9107)
  line L161 (38.0643, 31.9107) -> (18.7908, 20.291)
  arc A185 (15, 22.432) -> (18.7908, 20.291) centre (17.5, 22.432) ccw
  line L162 (15, 22.432) -> (15, 54.2597)
  arc A186 (15, 54.2597) -> (13.0261, 57.0788) centre (12, 54.2597) ccw
  line L163 (13.0261, 57.0788) -> (5.8285, 59.6985)
  arc A187 (5.8285, 59.6985) -> (4.1184, 60) centre (4.1184, 55) ccw
  circle A188 centre (18.0312, 0) radius 1.075
  circle A189 centre (-18.0312, 0) radius 1.075
  circle A190 centre (0, 18.0312) radius 1.075
  circle A191 centre (0, -18.0312) radius 1.075
  circle A192 centre (18.0312, 0) radius 2.25
  circle A193 centre (-18.0312, 0) radius 2.25
  circle A194 centre (0, 18.0312) radius 2.25
  circle A195 centre (0, -18.0312) radius 2.25
  dimension "d359" = 4.5
  dimension "d360" = 4.5
  dimension "d361" = 4.5
  dimension "d362" = 4.5
  constraint concentric A188 A192
  constraint concentric A189 A193
  constraint concentric A190 A194
  constraint concentric A118 A195
  measures "d359" diameter of A192
  measures "d360" diameter of A193
  measures "d361" diameter of A194
  measures "d362" diameter of A195
extrude "Extrude15" add sketch "Sketch7" along normal blind 3 contours A192 | A193 | A194 | A195 bodies 1
sketch "Sketch8" plane through (-13.75, 0, 0) normal (-1, 0, 0) x (0, -1, 0)
  arc A0 (-62.912, 15.0042) -> (-62.7914, 14.0886) centre (-61.9723, 14.6622) ccw
  line L0 (-62.912, 15.0042) -> (-59.5027, 24.371)
  arc A1 (-58.8395, 24.99) -> (-59.5027, 24.371) centre (-58.563, 24.029) ccw
  line L1 (-58.8395, 24.99) -> (-55.247, 26.0237)
  arc A2 (-53.9705, 25.0627) -> (-55.247, 26.0237) centre (-54.9705, 25.0627) ccw
  line L2 (-53.9705, 25.0627) -> (-53.9705, 8.5)
  arc A3 (-54.9705, 7.5) -> (-53.9705, 8.5) centre (-54.9705, 8.5) ccw
  line L3 (-54.9705, 7.5) -> (-57.6574, 7.5)
  arc A4 (-58.4766, 7.9264) -> (-57.6574, 7.5) centre (-57.6574, 8.5) ccw
  line L4 (-58.4766, 7.9264) -> (-62.7914, 14.0886)
  arc A5 (-50.4705, 8.5) -> (-49.4705, 7.5) centre (-49.4705, 8.5) ccw
  line L5 (-50.4705, 8.5) -> (-50.4705, 23.6889)
  arc A6 (-49.1285, 24.6286) -> (-50.4705, 23.6889) centre (-49.4705, 23.6889) ccw
  line L6 (-49.1285, 24.6286) -> (-38.4432, 20.7395)
  arc A7 (-37.7852, 19.7998) -> (-38.4432, 20.7395) centre (-38.7852, 19.7998) ccw
  line L7 (-37.7852, 19.7998) -> (-37.7852, 16.6911)
  arc A8 (-37.8193, 16.4323) -> (-37.7852, 16.6911) centre (-38.7852, 16.6911) ccw
  line L8 (-37.8193, 16.4323) -> (-39.119, 11.5817)
  arc A9 (-39.3778, 11.1334) -> (-39.119, 11.5817) centre (-40.0849, 11.8405) ccw
  line L9 (-39.3778, 11.1334) -> (-42.7183, 7.7929)
  arc A10 (-43.4254, 7.5) -> (-42.7183, 7.7929) centre (-43.4254, 8.5) ccw
  line L10 (-43.4254, 7.5) -> (-49.4705, 7.5)
  arc A11 (-66.646, 14.9783) -> (-66.4049, 13.1472) centre (-64.7666, 14.2943) ccw
  line L11 (-66.4049, 13.1472) -> (-60.5972, 4.8528)
  arc A12 (-60.5972, 4.8528) -> (-58.9589, 4) centre (-58.9589, 6) ccw
  line L12 (-58.9589, 4) -> (-54.9589, 4)
  line L13 (-54.9589, 4) -> (-54.9589, 0)
  line L14 (-54.9589, 0) -> (-43.3899, 0)
  line L15 (-43.3899, 0) -> (-43.3899, 4)
  line L16 (-43.3899, 4) -> (-42.3899, 4)
  arc A13 (-42.3899, 4) -> (-40.9757, 4.5858) centre (-42.3899, 6) ccw
  line L17 (-40.9757, 4.5858) -> (-36.4293, 9.1322)
  arc A14 (-36.4293, 9.1322) -> (-35.9116, 10.0288) centre (-37.8435, 10.5464) ccw
  line L18 (-35.9116, 10.0288) -> (-32.168, 24)
  line L19 (-32.168, 24) -> (-32.168, 26)
  line L20 (-32.168, 26) -> (-36.168, 26)
  line L21 (-36.168, 26) -> (-36.168, 24)
  line L22 (-36.168, 24) -> (-37.168, 24)
  line L23 (-37.168, 24) -> (-53.2322, 29.8469)
  arc A15 (-53.2322, 29.8469) -> (-54.4692, 29.8895) centre (-53.9162, 27.9675) ccw
  line L24 (-54.4692, 29.8895) -> (-61.0301, 28.0017)
  arc A16 (-61.0301, 28.0017) -> (-62.3565, 26.7637) centre (-60.4771, 26.0797) ccw
  line L25 (-62.3565, 26.7637) -> (-66.646, 14.9783)
  circle A17 centre (-47.1705, 15.3) radius 1
  arc A18 (-47.1998, 12.3001) -> (-47.1705, 18.3) centre (-47.1705, 15.3) ccw
  line L26 (-47.1705, 18.3) -> (-49.4705, 18.3)
  line L27 (-47.1998, 12.3001) -> (-49.4608, 12.3222)
  line L28 (-50.4705, 19.3) -> (-50.4705, 23.6889)
  line L29 (-50.4705, 11.3223) -> (-50.4705, 8.5)
  arc A19 (-50.4705, 19.3) -> (-49.4705, 18.3) centre (-49.4705, 19.3) ccw
  arc A20 (-49.4608, 12.3222) -> (-50.4705, 11.3223) centre (-49.4705, 11.3223) ccw
  dimension "d365" = 2
  dimension "d366" = 3.3
  dimension "d367" = 7.8
  dimension "d368" = 3
  dimension "d369" = 1
  constraint coincident A17.centre A18.centre
  constraint tangent A18 L26
  constraint perpendicular L5 L26
  constraint tangent A18 L27
  constraint coincident L5.end A6.end
  constraint coincident A5.start L5.start
  constraint tangent L26 A19
  constraint tangent L28 A19
  constraint tangent L27 A20
  constraint tangent L29 A20
  constraint equal A19 A20
  measures "d365" diameter of A17
  measures "d366" distance of L5 A17.centre
  measures "d367" distance of L10 A17.centre
  measures "d368" radius of A18
  measures "d369" radius of A19
extrude "Extrude16" add sketch "Sketch8" against normal blind 2.5 contours L5 A18 L26 L27 A19 A20 bodies 3
extrude "Extrude17" add sketch "Sketch8" against normal blind 2.5 from surface at -25 contours L5 A18 L26 L27 A19 A20 bodies 4